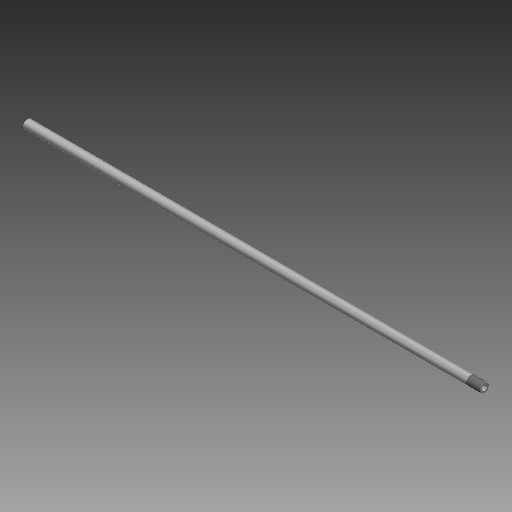
# Autodesk Inventor part: Shaft
Saved by Autodesk Inventor 2019.4 (Build 234330000, 330)
## iProperties
Created: 2020-01-09
Part Number: Shaft
Material: Steel
Document SubType Name: Modeling
Designer: Mark
Mass: 1559.78 g
Surface Area: 1004.16 cm^2
Volume: 198.698 cm^3
Density: 7.85 g/cm^3
Appearance: Steel
CustomPartVersion: 1
Length: 1000.000 mm
Author: Mark
Autodesk Inventor part; units mm, degrees
ref_plane "Start Plane" through (0, 0, 0) normal (1, 0, 0) x (0, 1, 0)
ref_plane "XZ Plane" through (0, 0, 0) normal (0, 1, 0) x (-1, 0, 0)
ref_plane "XY Plane" through (0, 0, 0) normal (0, 0, 1) x (1, 0, 0)
sketch "Main Sketch" plane through (0, 0, 0) normal (0, 0, 1) x (1, 0, 0)
  line L0 (0, 0) -> (1000, 0)
  line L1 (0, 5) -> (0, 10)
  line L2 (0, 10) -> (970, 10)
  line L3 (0, 5) -> (30, 5)
  line L4 (1000, 10) -> (1000, 6)
  line L5 (970, 10) -> (1000, 10)
  line L6 (30, 5) -> (30, 6)
  line L7 (1000, 6) -> (30, 6)
  dimension "d3" = 20
  dimension "d11" = 10
  dimension "d32" = 20
  dimension "d58" = 12
  constraints: 16 end point, 3 horizontal, 3 vertical
  measures "d3" diameter of L2 L0
  measures "d11" diameter of L3 L0
  measures "d32" diameter of L5 L0
  measures "d58" diameter of L7 L0
revolve "Revolution1" add sketch "Main Sketch" angle 360 about axis through (0, 0, 0) along (1, 0, 0)
thread "Thread18" size "TR20x2" class "7e" standard "ISO Metric Trapezoidal Threads" length 30
chamfer "Chamfer13" distance 0.6 angle 45 1 edges at (1000, -10, 0)
thread "Thread15" size "TR12x2" class "7H" standard "ISO Metric Trapezoidal Threads" length 30
chamfer "Chamfer11" distance 0.3 angle 45 1 edges at (30, -5, 0)
equation "\"Length\" = 1000"
body "Solid1"
